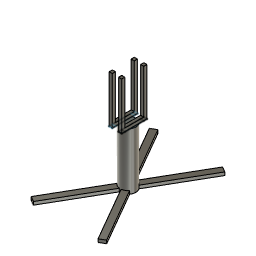
Test Stand (Autodesk Fusion 360 design; units mm, degrees)
Autodesk Fusion 360 part; units mm, degrees
sketch "Sketch1" plane through (0, 0, 0) normal (0, 0, 1) x (1, 0, 0)
  circle A0 centre (0, 0) radius 2.5
  line L0 (0.2796, 2.4843) -> (10.2796, 19.8048)
  line L1 (10.2796, 19.8048) -> (12.0117, 18.8048)
  line L2 (12.0117, 18.8048) -> (2.0117, 1.4843)
  line L3 (-0.2796, 2.4843) -> (-10.2796, 19.8048)
  line L4 (-10.2796, 19.8048) -> (-12.0117, 18.8048)
  line L5 (-12.0117, 18.8048) -> (-2.0117, 1.4843)
  line L6 (-2.0117, -1.4843) -> (-12.0117, -18.8048)
  line L7 (-12.0117, -18.8048) -> (-10.2796, -19.8048)
  line L8 (-10.2796, -19.8048) -> (-0.2796, -2.4843)
  line L9 (2.0117, -1.4843) -> (12.0117, -18.8048)
  line L10 (12.0117, -18.8048) -> (10.2796, -19.8048)
  line L11 (10.2796, -19.8048) -> (0.2796, -2.4843)
  line L12 (20, 0) -> (16, 0)
  dimension "d1" = 5
  dimension "d3" = 2
  dimension "d4" = 20
  dimension "d6" = 2
  dimension "d7" = 20
  dimension "d8" = 20
  dimension "d9" = 20
  dimension "d11" = 2
  dimension "d12" = 20
  dimension "d13" = 20
  dimension "d14" = 2
  dimension "d16" = 20
  dimension "d17" = 20
  dimension "d18" = 120
  dimension "d19" = 120
  dimension "d20" = 60
  dimension "d21" = 60
  constraint coincident A0.centre origin
  constraint coincident A0 L0.start
  constraint perpendicular L0 L1
  constraint coincident A0 L2.end
  constraint perpendicular L1 L2
  constraint coincident A0 L3.start
  constraint perpendicular L3 L4
  constraint coincident A0 L5.end
  constraint perpendicular L4 L5
  constraint coincident A0 L6.start
  constraint perpendicular L6 L7
  constraint coincident A0 L8.end
  constraint perpendicular L7 L8
  constraint coincident A0 L9.start
  constraint perpendicular L9 L10
  constraint coincident A0 L11.end
  constraint perpendicular L10 L11
  constraint horizontal L12
  measures "d1" diameter of A0
  measures "d3" distance of L0.end L1.end
  measures "d4" distance of L1.end L2.end
  measures "d6" distance of L3.end L4.end
  measures "d7" distance of L4.end L5.end
  measures "d8" distance of L3.start L3.end
  measures "d9" distance of L0.start L0.end
  measures "d11" distance of L6.end L7.end
  measures "d12" distance of L6.start L6.end
  measures "d13" distance of L7.end L8.end
  measures "d14" distance of L9.end L10.end
  measures "d16" distance of L9.start L9.end
  measures "d17" distance of L10.end L11.end
  measures "d18" angle of L5 L6
  measures "d19" angle of L2 L9
  measures "d20" angle of L0 L3
  measures "d21" angle of L2 L12
extrude "Extrude1" add sketch "Sketch1" along normal blind 1 contours A0 L0 L1 L2 | A0 L9 L10 L11 | A0 L3 L4 L5 | A0 L6 L7 L8 makes body 1 at (7.8471, 13.5916, 0) makes body 2 at (7.8471, -13.5916, 0) makes body 3 at (-7.8471, 13.5916, 0) makes body 4 at (-7.8471, -13.5916, 0)
extrude "Extrude2" add sketch "Sketch1" along normal blind 18 contours A0 bodies 1 2 3 4
sketch "Sketch2" plane through (0, 0, 18) normal (0, 0, 1) x (-1, 0, 0)
  circle A0 centre (0, 0) radius 2.5
  line L0 (-2, -4) -> (-1, -4)
  line L1 (-1, -4) -> (-1, 4)
  line L2 (-1, 4) -> (-2, 4)
  line L3 (-2, 4) -> (-2, -4)
  line L4 (2, -4) -> (1, -4)
  line L5 (1, -4) -> (1, 4)
  line L6 (1, 4) -> (2, 4)
  line L7 (2, 4) -> (2, -4)
  line L8 (-2, -3) -> (-1, -3)
  line L9 (-2, 3) -> (-1, 3)
  line L10 (1, -3) -> (2, -3)
  line L11 (1, 3) -> (2, 3)
  dimension "d26" = 8
  dimension "d27" = 8
  dimension "d30" = 1
  dimension "d31" = 1
  dimension "d32" = 2
  dimension "d33" = 4
  dimension "d34" = 1
  dimension "d35" = 1
  dimension "d36" = 1
  dimension "d37" = 1
  dimension "d40" = 1
  constraint horizontal L0
  constraint vertical L1
  constraint horizontal L2
  constraint vertical L3
  constraint horizontal L4
  constraint vertical L5
  constraint horizontal L6
  constraint vertical L7
  constraint coincident L3 L8.start
  constraint coincident L1 L8.end
  constraint perpendicular L1 L8
  constraint coincident L3 L9.start
  constraint coincident L1 L9.end
  constraint perpendicular L1 L9
  constraint coincident L5 L10.start
  constraint coincident L7 L10.end
  constraint perpendicular L7 L10
  constraint coincident L5 L11.start
  constraint coincident L7 L11.end
  constraint perpendicular L7 L11
  measures "d26" distance of L0.start L2.end
  measures "d27" distance of L4.start L6.end
  measures "d30" distance of L0.start L0.end
  measures "d31" distance of L4.start L4.end
  measures "d32" distance of L1 L5
  measures "d33" distance of A0.centre L2
  measures "d34" distance of L4 L10
  measures "d35" distance of L6 L11
  measures "d36" distance of L2 L9
  measures "d37" distance of L0 L8
  measures "d40" distance of A0.centre L1
extrude "Extrude3" add sketch "Sketch2" along normal blind 1 contours A0 L5 L7 | A0 L5 L7 L11 | A0 L5 L7 L10 | A0 L1 L3 | A0 L1 L3 L9 | A0 L1 L3 L8 bodies 1
extrude "Extrude4" add sketch "Sketch2" along normal blind 15 contours L5 L6 L7 L11 | L4 L5 L7 L10 | L1 L2 L3 L9 | L0 L1 L3 L8 bodies 1
